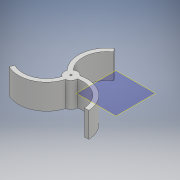
# Autodesk Inventor part: pump_impeller_rev_2
Saved by Autodesk Inventor 2017 (Build 210142000, 142)
## iProperties
Created: 2016-12-23
Part Number: pump_impeller_rev_2
Material: Generic
Document SubType Name: Modeling
Designer: Ali
Density: 1 g/cm^3
Appearance: Default
Author: Ali
Autodesk Inventor part; units mm, degrees
ref_plane "YZ Plane" through (0, 0, 0) normal (1, 0, 0) x (0, 1, 0)
ref_plane "XZ Plane" through (0, 0, 0) normal (0, 1, 0) x (-1, 0, 0)
ref_plane "XY Plane" through (0, 0, 0) normal (0, 0, 1) x (1, 0, 0)
ref_plane "Work Plane4" through (21.2718, 3.7508, -2.4) normal (0, 0, -1) x (-1, 0, 0)
sketch "Sketch5" plane through (21.2718, 3.7508, -2.4) normal (0, 0, -1) x (-1, 0, 0)
  arc A0 (24.639, -2.4773) -> (21.9352, 21.2492) centre (13.3117, 8.2492) ccw
  arc A1 (23.0748, -0.6348) -> (20.6085, 19.2492) centre (13.3118, 8.2492) ccw
  arc A2 (23.0687, -6.8701) -> (24.639, -2.4773) centre (21.2719, -3.7507) ccw
  arc A3 (23.0687, -6.8701) -> (41.5221, -14.6763) centre (35.6441, -2.8572) ccw
  line L0 (41.5221, -14.6763) -> (42.5908, -16.8253)
  arc A4 (20.691, -7.3035) -> (42.5908, -16.8253) centre (35.6441, -2.8572) ccw
  arc A5 (17.672, -3.7474) -> (20.691, -7.3035) centre (21.2719, -3.7507) ccw
  arc A6 (18.4854, -1.4715) -> (-0.7105, -15.6763) centre (14.8594, -16.6442) ccw
  arc A7 (23.0748, -0.6348) -> (18.4854, -1.4715) centre (21.2719, -3.7507) ccw
  arc A8 (17.672, -3.7474) -> (1.6849, -15.8253) centre (14.8595, -16.6443) ccw
  line L1 (1.6849, -15.8253) -> (-0.7105, -15.6763)
  line L2 (20.6085, 19.2492) -> (21.9352, 21.2492)
  point P0 (21.2718, -3.7508)
  dimension "d11" = 3.5999
  dimension "d13" = 13.2001
  dimension "d14" = 15.6002
  dimension "d15" = 13.2
  dimension "d16" = 15.5999
  dimension "d17" = 13.2001
  dimension "d18" = 15.6001
  constraints: 18 point on circle, 9 centre point, 6 end point
  measures "d11" radius of A7
  measures "d13" radius of A1
  measures "d14" radius of A0
  measures "d15" radius of A8
  measures "d16" radius of A6
  measures "d17" radius of A3
  measures "d18" radius of A4
extrude "Extrusion2" add sketch "Sketch5" along normal blind 14
sketch "Sketch6" plane through (21.2718, 3.7508, -2.4) normal (0, 0, 1) x (1, 0, 0)
  circle A0 centre (-21.2718, -3.7508) radius 1.5
  dimension "d21" = 3
  constraints: 1 centre point, 1 coincident
  measures "d21" diameter of A0
hole "Hole1" at (0, 0, -2.4) direction (0, 0, -1) diameter 1 depth 14 tip angle 118
body "Solid4"
